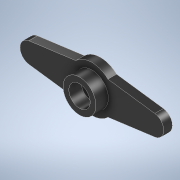
# Autodesk Inventor part: attachment_real
Saved by Autodesk Inventor 2022 (Build 260153000, 153)
## iProperties
Created: 2022-02-14
Part Number: attachment_real
Material: Nylon 6/6
Document SubType Name: Modeling
Designer: juanp
Density: 1.13 g/cm^3
Appearance: Nylon 6
Author: juanp
Autodesk Inventor part; units mm, degrees
ref_plane "YZ Plane" through (0, 0, 0) normal (1, 0, 0) x (0, 1, 0)
ref_plane "XZ Plane" through (0, 0, 0) normal (0, 1, 0) x (-1, 0, 0)
ref_plane "XY Plane" through (0, 0, 0) normal (0, 0, 1) x (1, 0, 0)
sketch "Sketch1" plane through (0, 0, 0) normal (0, 0, 1) x (1, 0, 0)
  circle A0 centre (0, 0) radius 6.15
  line L0 (-4.2968, 4.4) -> (-16.8146, 2.7257)
  arc A1 (-16.8146, 2.7257) -> (-16.8146, -2.7257) centre (-16.45, 0) ccw
  line L1 (-16.8146, -2.7257) -> (-4.2968, -4.4)
  line L2 (4.2968, -4.4) -> (16.8146, -2.7257)
  arc A2 (16.8146, -2.7257) -> (16.8146, 2.7257) centre (16.45, 0) ccw
  line L3 (16.8146, 2.7257) -> (4.2968, 4.4)
  line L4 (-4.2968, -4.4) -> (4.2968, -4.4) construction
  line L5 (-4.2968, 4.4) -> (4.2968, 4.4) construction
  line L6 (-19.2, 0) -> (19.2, 0) construction
  dimension "d0" = 12.3
  dimension "d1" = 8.8
  dimension "d2" = 38.4
  dimension "d3" = 2.75
  constraints: 14 end point, 10 point on circle, 4 equal length, 4 tangent, 3 centre point, 2 horizontal, 1 coincident, 1 equal radius
  measures "d0" diameter of A0
  measures "d1" distance between parallel lines of L5 L4
  measures "d2" distance of L6.start L6.end
  measures "d3" radius of A2
extrude "Extrusion1" add sketch "Sketch1" along normal blind 2.3
sketch "Sketch2" plane through (0, 0, 2.3) normal (0, 0, 1) x (1, 0, 0)
  circle A0 centre (0, 0) radius 4.4
  circle A1 centre (0, 0) radius 2.85
  dimension "d6" = 8.8
  dimension "d7" = 5.7
  constraints: 2 centre point, 2 coincident
  measures "d6" diameter of A0
  measures "d7" diameter of A1
extrude "Extrusion2" add sketch "Sketch2" along normal blind 3.3
body "Solid1"
